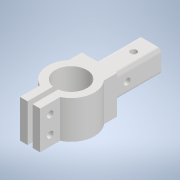
# Autodesk Inventor part: 5_Connettore_sup_inf
Saved by Autodesk Inventor 2020 (Build 240168000, 168)
## iProperties
Created: 2019-10-13
Part Number: 5_Connettore_sup_inf
Material: Generico
Document SubType Name: Modeling
Designer: socci
Density: 1 g/cm^3
Appearance: Default
Author: socci
Autodesk Inventor part; units mm, degrees
ref_plane "YZ Plane" through (0, 0, 0) normal (1, 0, 0) x (0, 1, 0)
ref_plane "XZ Plane" through (0, 0, 0) normal (0, 1, 0) x (-1, 0, 0)
ref_plane "XY Plane" through (0, 0, 0) normal (0, 0, 1) x (1, 0, 0)
sketch "Schizzo1" plane through (0, 0, 0) normal (0, 0, 1) x (1, 0, 0)
  line L0 (9, 6) -> (9, -6)
  line L1 (6, -9) -> (-6, -9)
  line L2 (-9, -6) -> (-9, 6)
  line L3 (-6, 9) -> (6, 9)
  arc A0 (-6, 9) -> (-9, 6) centre (-6, 6) ccw
  arc A1 (-9, -6) -> (-6, -9) centre (-6, -6) ccw
  arc A2 (6, -9) -> (9, -6) centre (6, -6) ccw
  arc A3 (9, 6) -> (6, 9) centre (6, 6) ccw
  point P0 (0, 0)
  point P1 (0, 0)
  point P2 (9, 9)
  point P3 (9, -9)
  point P4 (-9, -9)
  point P5 (-9, 9)
  dimension "d0" = 18
  dimension "d72" = 3
  constraints: 8 end point, 8 point on circle, 8 point on line, 8 tangent, 4 centre point, 3 equal radius, 1 coincident, 9 other
  measures "d0" distance of point (9, 9) point (9, -9)
  measures "d72" radius of A0
extrude "Estrusione1" add sketch "Schizzo1" against normal blind 40
sketch "Schizzo2" plane through (0, 0, 0) normal (0, 0, 1) x (1, 0, 0)
  line L0 (18.5, -15) -> (-18.5, -15)
  line L1 (-18.5, -15) -> (-18.5, 15)
  line L2 (-18.5, 15) -> (18.5, 15)
  line L3 (18.5, 15) -> (18.5, -15)
  line L4 (18.5, -15) -> (-18.5, 15) construction
  line L5 (-18.5, -15) -> (18.5, 15) construction
  point P0 (0, 0)
  dimension "d3" = 30
  dimension "d4" = 37
  constraints: 12 end point, 3 midpoint, 2 parallel, 1 horizontal, 1 perpendicular
  measures "d3" distance of L0.end L1.end
  measures "d4" distance of L1.end L2.end
extrude "Estrusione2" add sketch "Schizzo2" along normal blind 50
sketch "Schizzo3" plane through (-18.5, 15, 0) normal (0, 1, 0) x (1, 0, 0)
  line L0 (18.5, 0) -> (18.5, -22.5)
  line L1 (18.5, 0) -> (41, 0) construction
  circle A0 centre (18.5, -22.5) radius 12.5
  dimension "d7" = 22.5
  dimension "d8" = 90
  dimension "d9" = 25
  constraints: 4 end point, 1 centre point, 1 coincident, 1 horizontal, 1 perpendicular, 1 vertical
  measures "d7" distance of L0.start L0.end
  measures "d8" angle of L0 L1
  measures "d9" diameter of A0
extrude "Estrusione3" cut sketch "Schizzo3" against normal blind 30
sketch "Schizzo4" plane through (-18.5, 15, 0) normal (0, 1, 0) x (1, 0, 0)
  circle A0 centre (18.5, -22.5) radius 12.5 projected
  line L0 (18.5, -22.5) -> (18.5, -34.5)
  line L1 (18.5, -34.5) -> (15, -34.5)
  line L2 (18.5, -34.5) -> (22, -34.5)
  line L3 (0, -50) -> (37, -50) projected
  line L4 (18.5, -50) -> (20.5, -50)
  line L5 (18.5, -50) -> (20.5, -50) construction
  line L6 (20.5, -50) -> (20.5, -34.5)
  line L7 (18.5, -50) -> (16.5, -50)
  line L8 (16.5, -50) -> (20.5, -50)
  line L9 (20.5, -50) -> (20.5, -34.5)
  line L10 (20.5, -34.5) -> (16.5, -34.5)
  line L11 (16.5, -34.5) -> (16.5, -50)
  point P0 (18.5, 0)
  point P1 (16.5, -34.839)
  point P2 (20.5, -34.839)
  dimension "d12" = 12
  dimension "d13" = 2
  dimension "d14" = 0
  dimension "d15" = 2
  constraints: 22 end point, 3 collinear, 3 perpendicular, 3 point on line, 2 parallel, 2 point on circle, 1 horizontal, 1 midpoint, 1 vertical
  measures "d12" distance of L0.start L0.end
  measures "d13" distance of L4.start L4.end
  measures "d14" distance between parallel lines of L4 L5
  measures "d15" distance of L4.start L7.end
extrude "Estrusione4" cut sketch "Schizzo4" against normal blind 30 contours A0 L6 L3 L11
sketch "Schizzo5" plane through (-18.5, 15, 0) normal (0, 1, 0) x (1, 0, 0)
  arc A0 (20.5, -34.839) -> (16.5, -34.839) centre (18.5, -22.5) ccw projected
  circle A1 centre (18.5, -22.5) radius 18.5
  line L0 (20.5, -50) -> (20.5, -34.839) projected
  line L1 (20.5, -50) -> (26.5, -50)
  line L2 (37, -50) -> (20.5, -50) projected
  line L3 (26.5, -50) -> (26.5, -39.1808)
  line L4 (37, 0) -> (37, -50) projected
  line L5 (26.5, -50) -> (37, -50)
  line L6 (37, -50) -> (37, -22.5)
  point P0 (18.5, 0)
  dimension "d18" = 37
  dimension "d19" = 6
  constraints: 8 end point, 2 perpendicular, 2 point on circle, 2 point on line, 1 centre point, 1 coincident
  measures "d18" diameter of A1
  measures "d19" distance of L0.start L1.end
extrude "Estrusione5" cut sketch "Schizzo5" against normal blind 30 contours A1 L4 L2 L3
sketch "Schizzo6" plane through (-18.5, 15, 0) normal (0, 1, 0) x (1, 0, 0)
  line L0 (16.5, -50) -> (0, -50) projected
  line L1 (16.5, -50) -> (10.5, -50)
  arc A0 (20.5, -34.839) -> (16.5, -34.839) centre (18.5, -22.5) ccw projected
  circle A1 centre (18.5, -22.5) radius 18.5
  line L2 (0, 0) -> (0, -50) projected
  line L3 (10.5, -50) -> (0, -50)
  line L4 (0, -50) -> (0, -22.5)
  line L5 (10.5, -50) -> (10.5, -39.1808)
  line L6 (10.5, -50) -> (21.3192, -50) construction
  point P0 (18.5, 0)
  dimension "d22" = 6
  dimension "d23" = 37
  dimension "d24" = 90
  constraints: 10 end point, 2 horizontal, 2 point on circle, 2 point on line, 1 centre point, 1 coincident, 1 perpendicular
  measures "d22" distance of L0.start L1.end
  measures "d23" diameter of A1
  measures "d24" angle of L6 L5
extrude "Estrusione6" cut sketch "Schizzo6" against normal blind 30 contours L0 L2 A1 L5
sketch "Schizzo7" plane through (-18.5, 15, 0) normal (0, 1, 0) x (1, 0, 0)
  arc A0 (20.5, -34.839) -> (16.5, -34.839) centre (18.5, -22.5) ccw projected
  circle A1 centre (18.5, -22.5) radius 18.5
  line L0 (9.5, 0) -> (9.5, 40) projected
  line L1 (9.5, 0) -> (0, 0)
  line L2 (0, 0) -> (0, -22.5)
  line L3 (18.5, 0) -> (4.5, 0)
  line L4 (18.5, 0) -> (32.5, 0) construction
  line L5 (4.5, 0) -> (4.5, -10.4066)
  dimension "d27" = 37
  dimension "d28" = 14
  dimension "d29" = 180
  dimension "d30" = 90
  constraints: 10 end point, 2 collinear, 2 point on circle, 1 centre point, 1 coincident, 1 horizontal, 1 perpendicular, 1 tangent
  measures "d27" diameter of A1
  measures "d28" distance of L3.start L3.end
  measures "d29" angle of L3 L4
  measures "d30" angle of L5 L3
extrude "Estrusione7" cut sketch "Schizzo7" against normal blind 30 contours A1 L2 L1 L5
sketch "Schizzo8" plane through (0, 15, 22.5) normal (0, 1, 0) x (1, 0, 0)
  line L0 (-6, 22.5) -> (6, 22.5) projected
  arc A0 (2, -12.339) -> (-2, -12.339) centre (0, 0) ccw projected
  circle A1 centre (0, 0) radius 18.5
  line L1 (0, 22.5) -> (14, 22.5)
  line L2 (0, 22.5) -> (14, 22.5) construction
  line L3 (14, 22.5) -> (14, 12.0934)
  line L4 (-14, 22.5) -> (18.5, 22.5) projected
  line L5 (14, 22.5) -> (18.5, 22.5)
  line L6 (18.5, 22.5) -> (18.5, 0)
  point P0 (-9, 22.5)
  point P1 (9, 22.5)
  dimension "d35" = 37
  dimension "d36" = 14
  dimension "d37" = 0
  dimension "d38" = 90
  constraints: 10 end point, 2 collinear, 2 horizontal, 2 point on circle, 1 centre point, 1 coincident, 1 perpendicular
  measures "d35" diameter of A1
  measures "d36" distance of L1.start L1.end
  measures "d37" distance between parallel lines of L1 L2
  measures "d38" angle of L1 L3
extrude "Estrusione8" cut sketch "Schizzo8" against normal blind 30 contours A1 L3 L4 L6
sketch "Schizzo10" plane through (0, 0, 50) normal (0, 0, 1) x (1, 0, 0)
  line L0 (-8, 15) -> (-8, -15) projected
  line L1 (-8, -15) -> (8.0102, -15)
  line L2 (8.0102, -15) -> (8.0102, 15)
  line L3 (8.0102, 15) -> (-8, 15)
  line L4 (-8, 15) -> (-8, -15)
  line L5 (-8, -15) -> (-2, -15) projected
  line L6 (2, 15) -> (2, -15) projected
  line L7 (-2, -15) -> (2, -15)
  line L8 (2, -15) -> (2, 15)
  line L9 (2, 15) -> (-2, 15)
  line L10 (-2, 15) -> (-2, -15)
  point P0 (0, 0)
  point P1 (-8, 15)
  constraints: 16 end point, 4 parallel, 4 perpendicular
extrude "Estrusione9" add sketch "Schizzo10" along normal blind 5 contours L3 L10 L1 L0 | L3 L2 L1 L6
sketch "Schizzo11" plane through (-8, -15, 39.1808) normal (-1, 0, 0) x (0, 0, 1)
  line L0 (15.8192, 0) -> (15.8192, 30) projected
  line L1 (15.8192, 15) -> (7.8192, 15)
  line L2 (7.8192, 15) -> (7.8192, 22)
  line L3 (7.8192, 15) -> (7.8192, 8)
  line L4 (10.8192, 0) -> (10.8192, 30) projected
  line L5 (7.8192, 15) -> (14.8192, 15) construction
  point P0 (-39.1808, 15)
  dimension "d43" = 8
  dimension "d44" = 7
  dimension "d45" = 7
  dimension "d46" = 90
  constraints: 8 end point, 2 horizontal, 1 midpoint, 1 parallel, 1 perpendicular, 1 vertical
  measures "d43" distance of L1.start L1.end
  measures "d44" distance of L1.end L2.end
  measures "d45" distance of L1.end L3.end
  measures "d46" angle of L3 L5
hole "Foro1" at (-8, 7, 47) at (-8, -7, 47) direction (1, 0, 0) diameter 5 end through all
sketch "Schizzo12" plane through (-9, -9, -40) normal (-1, 0, 0) x (0, 0, 1)
  line L0 (40, 9) -> (27, 9)
  line L1 (40, 9) -> (53, 9) construction
  dimension "d54" = 13
  dimension "d55" = 180
  constraints: 4 end point, 2 horizontal, 1 collinear
  measures "d54" distance of L0.start L0.end
  measures "d55" angle of L0 L1
hole "Foro2" at (-9, 0, -13) direction (1, 0, 0) diameter 5 end through all
sketch "Schizzo13" plane through (-9, 9, -40) normal (0, 1, 0) x (1, 0, 0)
  line L0 (15, 0) -> (3, 0) projected
  line L1 (9, 0) -> (9, -13)
  line L2 (9, 0) -> (22, 0) construction
  point P0 (9, -40)
  point P1 (18, 0)
  point P2 (0, 0)
  dimension "d63" = 13
  dimension "d64" = 90
  constraints: 4 end point, 1 horizontal, 1 midpoint, 1 perpendicular, 1 vertical
  measures "d63" distance of L1.start L1.end
  measures "d64" angle of L1 L2
hole "Foro3" at (0, 9, -27) direction (0, -1, 0) diameter 5 end through all
